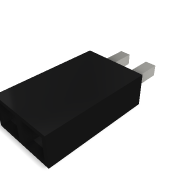
# Autodesk Inventor part: 2  female pin
Saved by Autodesk Inventor 2020 (Build 240168000, 168)
## iProperties
Created: 2018-03-11
Part Number: 2  female pin
Material: Generic
Document SubType Name: Modeling
Designer: Alex
Density: 1 g/cm^3
Appearance: Default
Author: Alex
Autodesk Inventor part; units mm, degrees
ref_plane "YZ Plane" through (0, 0, 0) normal (1, 0, 0) x (0, 1, 0)
ref_plane "XZ Plane" through (0, 0, 0) normal (0, 1, 0) x (-1, 0, 0)
ref_plane "XY Plane" through (0, 0, 0) normal (0, 0, 1) x (1, 0, 0)
sketch "Sketch1" plane through (0, 0, 0) normal (0, 0, 1) x (1, 0, 0)
  line L0 (1.27, -1.27) -> (-1.27, -1.27)
  line L1 (-1.27, -1.27) -> (-1.27, 1.27)
  line L2 (-1.27, 1.27) -> (1.27, 1.27)
  line L3 (1.27, 1.27) -> (1.27, -1.27)
  line L4 (1.27, -1.27) -> (-1.27, 1.27) construction
  line L5 (-1.27, -1.27) -> (1.27, 1.27) construction
  point P0 (0, 0)
  dimension "d0" = 2.54
  dimension "d1" = 2.54
  constraints: 12 end point, 2 midpoint, 2 parallel, 1 horizontal, 1 perpendicular
  measures "d0" distance of L1.end L2.end
  measures "d1" distance of L0.end L1.end
extrude "Extrusion1" add sketch "Sketch1" along normal blind 8.382
sketch "Sketch2" plane through (0, 0, 8.382) normal (0, 0, 1) x (1, 0, 0)
  line L0 (0.5715, 0.5715) -> (-0.5715, 0.5715)
  line L1 (-0.5715, 0.5715) -> (-0.5715, -0.5715)
  line L2 (-0.5715, -0.5715) -> (0.5715, -0.5715)
  line L3 (0.5715, -0.5715) -> (0.5715, 0.5715)
  line L4 (0.5715, 0.5715) -> (-0.5715, -0.5715) construction
  line L5 (-0.5715, 0.5715) -> (0.5715, -0.5715) construction
  point P0 (0, 0)
  dimension "d4" = 1.143
  constraints: 12 end point, 2 midpoint, 2 parallel, 2 perpendicular, 1 horizontal
  measures "d4" distance of L2.end L1.end
extrude "Extrusion2" cut sketch "Sketch2" against normal blind 6.35
chamfer "Chamfer1" distance 0.381 angle 45 4 edges at (0, 0.5715, 8.382) (-0.5715, 0, 8.382) (0, -0.5715, 8.382) (0.5715, 0, 8.382)
sketch "Sketch3" plane through (0, 0, 0) normal (0, 0, -1) x (-1, 0, 0)
  line L0 (0.4445, -0.4445) -> (-0.4445, -0.4445)
  line L1 (-0.4445, -0.4445) -> (-0.4445, 0.4445)
  line L2 (-0.4445, 0.4445) -> (0.4445, 0.4445)
  line L3 (0.4445, 0.4445) -> (0.4445, -0.4445)
  line L4 (0.4445, -0.4445) -> (-0.4445, 0.4445) construction
  line L5 (-0.4445, -0.4445) -> (0.4445, 0.4445) construction
  point P0 (0, 0)
  dimension "d10" = 0.889
  constraints: 12 end point, 2 midpoint, 2 parallel, 2 perpendicular, 1 horizontal
  measures "d10" distance of L1.end L2.end
extrude "Extrusion3" add sketch "Sketch3" along normal blind 3.302
chamfer "Chamfer2" distance 0.381 angle 45 4 edges at (0, 0.4445, -3.302) (-0.4445, 0, -3.302) (0, -0.4445, -3.302) (0.4445, 0, -3.302)
pattern_linear "Rectangular Pattern1" count 2 spacing 2.54 along (1, 0, 0) of "Extrusion1", "Extrusion2", "Chamfer1", "Extrusion3", "Chamfer2"
equation "\"d1\" = d0"
body "Solid1"
